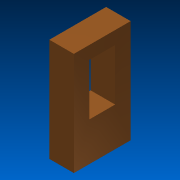
# Autodesk Inventor part: SPDT Toggle Switch Pin
Saved by Autodesk Inventor 2011 SP1 (Build 150282100, 282)
## iProperties
Created: 2011-11-07
Part Number: SPDT Toggle Switch Pin
Document SubType Name: Modeling
Designer: sdarley
Density: 1 g/cm^3
Author: sdarley
Autodesk Inventor part; units mm, degrees
ref_plane "YZ Plane" through (0, 0, 0) normal (1, 0, 0) x (0, 1, 0)
ref_plane "XZ Plane" through (0, 0, 0) normal (0, 1, 0) x (-1, 0, 0)
ref_plane "XY Plane" through (0, 0, 0) normal (0, 0, 1) x (1, 0, 0)
sketch "Sketch1" plane through (0, 0, 0) normal (0, 0, 1) x (1, 0, 0)
  line L0 (-0.5, 7) -> (-1.725, 7) projected
  line L1 (-13, 0.5) -> (-13, 6.5) projected
  line L2 (-11.275, 0) -> (-12.5, 0) projected
  line L3 (0, 0.5) -> (0, 6.5) projected
  line L4 (-12, 4.6) -> (-11.05, 4.6)
  line L5 (-11.05, 4.6) -> (-11.05, 2.4)
  line L6 (-11.05, 2.4) -> (-12, 2.4)
  line L7 (-12, 2.4) -> (-12, 4.6)
  arc A0 (-12.5, 7) -> (-13, 6.5) centre (-12.5, 6.5) ccw projected
  arc A1 (-13, 0.5) -> (-12.5, 0) centre (-12.5, 0.5) ccw projected
  line L8 (-11.275, 0) -> (-11.275, 0.5) projected
  line L9 (-11.275, 0.5) -> (-1.725, 0.5) projected
  line L10 (-1.725, 0.5) -> (-1.725, 0) projected
  line L11 (-0.5, 0) -> (-1.725, 0) projected
  arc A2 (-0.5, 0) -> (0, 0.5) centre (-0.5, 0.5) ccw projected
  arc A3 (0, 6.5) -> (-0.5, 7) centre (-0.5, 6.5) ccw projected
  line L12 (-1.725, 7) -> (-1.725, 6.5) projected
  line L13 (-1.725, 6.5) -> (-11.275, 6.5) projected
  line L14 (-11.275, 6.5) -> (-11.275, 7) projected
  line L15 (-11.275, 7) -> (-12.5, 7) projected
  point P0 (0, 0)
  point P1 (-13, 3.5)
  point P2 (-12, 3.5)
  dimension "d0" = 0.95
  dimension "d1" = 2.2
  constraints: 8 end point, 2 midpoint, 2 parallel, 1 horizontal, 1 horizontal alignment, 1 perpendicular
  measures "d0" distance between parallel lines of L5 L7
  measures "d1" distance between parallel lines of L6 L4
extrude "Extrusion1" add sketch "Sketch1" along normal blind 4 contours L4 L5 L6 L7
sketch "Sketch2" plane through (-11.05, 2.4, 0) normal (1, 0, 0) x (0, 0, -1)
  line L0 (-4, 2.2) -> (-4, 0) projected
  line L1 (0, 2.2) -> (0, 0) projected
  line L2 (-3.5, 1.6) -> (-1.5, 1.6)
  line L3 (-1.5, 1.6) -> (-1.5, 0.6)
  line L4 (-1.5, 0.6) -> (-3.5, 0.6)
  line L5 (-3.5, 0.6) -> (-3.5, 1.6)
  point P0 (0, -2.4)
  point P1 (0, 1.1)
  point P2 (-1.5, 1.1)
  dimension "d4" = 1
  dimension "d5" = 2
  dimension "d6" = 0.5
  constraints: 8 end point, 2 midpoint, 2 parallel, 1 horizontal, 1 horizontal alignment, 1 perpendicular
  measures "d4" distance between parallel lines of L4 L2
  measures "d5" distance between parallel lines of L5 L3
  measures "d6" distance between parallel lines of L0 L5
extrude "Extrusion2" cut sketch "Sketch2" against normal through all
body "Solid1"
